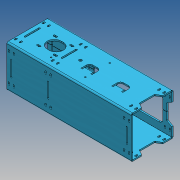
# Autodesk Inventor part: Pliegue Principal
Saved by Autodesk Inventor 2017 (Build 210142000, 142)
## iProperties
Part Number: Pliegue Principal
Material: Genérico
Document SubType Name: Chapa
Designer: Leo
Density: 1 g/cm^3
Appearance: Turquesa
Sheet Metal Rule: Por defecto
Sheet Metal Width: 355,000 mm
Sheet Metal Length: 458,387 mm
Sheet Metal Area: 162727,287 mm^2
Flat Pattern Width: 35.5 cm
Flat Pattern Length: 45.8387 cm
Flat Pattern Area: 1627.27 cm^2
Author: Leo
Autodesk Inventor part; units mm, degrees
ref_plane "YZ Plane" through (0, 0, 0) normal (1, 0, 0) x (0, 1, 0)
ref_plane "XZ Plane" through (0, 0, 0) normal (0, 1, 0) x (-1, 0, 0)
ref_plane "XY Plane" through (0, 0, 0) normal (0, 0, 1) x (1, 0, 0)
sketch "Boceto1" plane through (0, 0, 0) normal (0, 0, 1) x (1, 0, 0)
  circle A0 centre (0, 0) radius 4.805 construction
  circle A1 centre (0, 0) radius 22 construction
  circle A2 centre (72, 0) radius 50 construction
  line L0 (28.2, 28.2) -> (-28.2, 28.2) construction
  line L1 (-28.2, 28.2) -> (-28.2, -28.2) construction
  line L2 (-28.2, -28.2) -> (28.2, -28.2) construction
  line L3 (28.2, -28.2) -> (28.2, 28.2) construction
  line L4 (-8.5556, 20.2683) -> (52.5556, 46.0642) construction
  line L5 (52.5556, -46.0642) -> (-8.5556, -20.2683) construction
  line L6 (51.8, -14) -> (251.8, -14) construction
  line L7 (251.8, -14) -> (251.8, -56) construction
  line L8 (251.8, -56) -> (51.8, -56) construction
  line L9 (51.8, -56) -> (51.8, -14) construction
  circle A3 centre (72, 0) radius 4
  line L10 (-20.57, 21.07) -> (-26.57, 21.07)
  arc A4 (-26.57, 26.07) -> (-26.57, 21.07) centre (-26.57, 23.57) ccw
  line L11 (-26.57, 26.07) -> (-20.57, 26.07)
  arc A5 (-20.57, 21.07) -> (-20.57, 26.07) centre (-20.57, 23.57) ccw
  line L12 (20.57, -21.07) -> (26.57, -21.07)
  arc A6 (26.57, -26.07) -> (26.57, -21.07) centre (26.57, -23.57) ccw
  line L13 (26.57, -26.07) -> (20.57, -26.07)
  arc A7 (20.57, -21.07) -> (20.57, -26.07) centre (20.57, -23.57) ccw
  line L14 (20.57, 26.07) -> (26.57, 26.07)
  arc A8 (26.57, 21.07) -> (26.57, 26.07) centre (26.57, 23.57) ccw
  line L15 (26.57, 21.07) -> (20.57, 21.07)
  arc A9 (20.57, 26.07) -> (20.57, 21.07) centre (20.57, 23.57) ccw
  line L16 (-20.57, 23.57) -> (-26.57, 23.57) construction
  line L17 (20.57, 23.57) -> (26.57, 23.57) construction
  line L18 (48.6318, 0) -> (95.3682, 0) construction
  circle A10 centre (120.734, 35) radius 2
  circle A11 centre (120.734, -35) radius 2
  circle A12 centre (120.734, 35) radius 10 construction
  circle A13 centre (72, 0) radius 30 construction
  line L19 (119.667, 25.0571) -> (75.2009, 29.8287) construction
  line L20 (-78.2, 60) -> (276.8, 60)
  line L21 (276.8, 60) -> (276.8, -60)
  line L22 (276.8, -60) -> (-78.2, -60)
  line L23 (-78.2, -60) -> (-78.2, 60)
  circle A14 centre (23.266, -35) radius 2
  circle A15 centre (23.266, -35) radius 10 construction
  circle A16 centre (72, 0) radius 11 construction
  line L24 (-26.57, -21.07) -> (-20.57, -21.07)
  arc A17 (-20.57, -26.07) -> (-20.57, -21.07) centre (-20.57, -23.57) ccw
  line L25 (-20.57, -26.07) -> (-26.57, -26.07)
  arc A18 (-26.57, -21.07) -> (-26.57, -26.07) centre (-26.57, -23.57) ccw
  line L26 (-26.57, -23.57) -> (-20.57, -23.57) construction
  line L27 (-23.57, -23.57) -> (-23.57, 23.57) construction
  line L28 (23.57, 23.57) -> (23.57, -18.9602) construction
  line L29 (-23.57, 0) -> (23.57, 0) construction
  line L30 (-3, -20) -> (3, -20)
  arc A19 (3, -20) -> (3, 20) centre (3, 0) ccw
  line L31 (3, 20) -> (-3, 20)
  arc A20 (-3, 20) -> (-3, -20) centre (-3, 0) ccw
  line L32 (-67.9, 20.5) -> (-67.9, -20.5)
  arc A21 (-67.9, -20.5) -> (-63.5, -20.5) centre (-65.7, -20.5) ccw
  line L33 (-63.5, -20.5) -> (-63.5, 20.5)
  arc A22 (-63.5, 20.5) -> (-67.9, 20.5) centre (-65.7, 20.5) ccw
  line L34 (266.5, 20.5) -> (266.5, -20.5)
  arc A23 (262.1, -20.5) -> (266.5, -20.5) centre (264.3, -20.5) ccw
  line L35 (262.1, -20.5) -> (262.1, 20.5)
  arc A24 (266.5, 20.5) -> (262.1, 20.5) centre (264.3, 20.5) ccw
  line L36 (99.3, 60) -> (99.3, -60) construction
  line L37 (37.8, 20.5) -> (37.8, -20.5)
  arc A25 (37.8, -20.5) -> (42.2, -20.5) centre (40, -20.5) ccw
  line L38 (42.2, -20.5) -> (42.2, 20.5)
  arc A26 (42.2, 20.5) -> (37.8, 20.5) centre (40, 20.5) ccw
  line L39 (42.2, 0) -> (37.8, 0) construction
  line L40 (40, -20.5) -> (40, 20.5) construction
  line L41 (92.15, -19) -> (92.15, -3)
  arc A27 (101.15, 6) -> (92.15, -3) centre (101.15, -3) ccw
  line L42 (101.15, 6) -> (115.15, 6)
  arc A28 (124.15, -3) -> (115.15, 6) centre (115.15, -3) ccw
  line L43 (124.15, -3) -> (124.15, -19)
  line L44 (120.15, -19) -> (120.15, -3)
  arc A29 (120.15, -3) -> (115.15, 2) centre (115.15, -3) ccw
  line L45 (115.15, 2) -> (101.15, 2)
  arc A30 (101.15, 2) -> (96.15, -3) centre (101.15, -3) ccw
  line L46 (96.15, -3) -> (96.15, -19)
  line L47 (120.15, -19) -> (124.15, -19)
  line L48 (96.15, -19) -> (92.15, -19)
  circle A31 centre (108.15, -4) radius 1.5
  line L49 (120.15, -10) -> (96.15, -10) construction
  line L50 (152.15, 24.7694) -> (152.15, -40.3489) construction
  line L51 (212.15, -19) -> (212.15, -3)
  arc A32 (212.15, -3) -> (203.15, 6) centre (203.15, -3) ccw
  line L52 (203.15, 6) -> (189.15, 6)
  arc A33 (189.15, 6) -> (180.15, -3) centre (189.15, -3) ccw
  line L53 (180.15, -3) -> (180.15, -19)
  line L54 (184.15, -19) -> (184.15, -3)
  arc A34 (189.15, 2) -> (184.15, -3) centre (189.15, -3) ccw
  line L55 (189.15, 2) -> (203.15, 2)
  arc A35 (208.15, -3) -> (203.15, 2) centre (203.15, -3) ccw
  line L56 (208.15, -3) -> (208.15, -19)
  line L57 (184.15, -19) -> (180.15, -19)
  line L58 (208.15, -19) -> (212.15, -19)
  circle A36 centre (196.15, -4) radius 1.5
  line L59 (184.15, -10) -> (208.15, -10) construction
  line L60 (-72.9, 44.2) -> (-72.9, 35.8) construction
  line L61 (-75.1, 42) -> (-75.1, 38)
  line L62 (-70.7, 38) -> (-70.7, 42)
  arc A37 (-70.7, 42) -> (-75.1, 42) centre (-72.9, 42) ccw
  arc A38 (-75.1, 38) -> (-70.7, 38) centre (-72.9, 38) ccw
  line L63 (-58.5, 44.2) -> (-58.5, 35.8) construction
  line L64 (-60.7, 42) -> (-60.7, 38)
  line L65 (-56.3, 38) -> (-56.3, 42)
  arc A39 (-56.3, 42) -> (-60.7, 42) centre (-58.5, 42) ccw
  arc A40 (-60.7, 38) -> (-56.3, 38) centre (-58.5, 38) ccw
  line L66 (-65.7, 20.5) -> (-65.7, -20.5) construction
  line L67 (-72.9, -44.2) -> (-72.9, -35.8) construction
  line L68 (-75.1, -42) -> (-75.1, -38)
  line L69 (-70.7, -38) -> (-70.7, -42)
  arc A41 (-75.1, -42) -> (-70.7, -42) centre (-72.9, -42) ccw
  arc A42 (-70.7, -38) -> (-75.1, -38) centre (-72.9, -38) ccw
  line L70 (-58.5, -44.2) -> (-58.5, -35.8) construction
  line L71 (-60.7, -42) -> (-60.7, -38)
  line L72 (-56.3, -38) -> (-56.3, -42)
  arc A43 (-60.7, -42) -> (-56.3, -42) centre (-58.5, -42) ccw
  arc A44 (-56.3, -38) -> (-60.7, -38) centre (-58.5, -38) ccw
  line L73 (273.7, 42) -> (273.7, 38)
  line L74 (269.3, 38) -> (269.3, 42)
  arc A45 (273.7, 42) -> (269.3, 42) centre (271.5, 42) ccw
  arc A46 (269.3, 38) -> (273.7, 38) centre (271.5, 38) ccw
  line L75 (259.3, 42) -> (259.3, 38)
  line L76 (254.9, 38) -> (254.9, 42)
  arc A47 (259.3, 42) -> (254.9, 42) centre (257.1, 42) ccw
  arc A48 (254.9, 38) -> (259.3, 38) centre (257.1, 38) ccw
  arc A49 (273.7, -38) -> (269.3, -38) centre (271.5, -38) ccw
  arc A50 (259.3, -38) -> (254.9, -38) centre (257.1, -38) ccw
  line L77 (259.3, -42) -> (259.3, -38)
  line L78 (269.3, -38) -> (269.3, -42)
  line L79 (254.9, -38) -> (254.9, -42)
  arc A51 (254.9, -42) -> (259.3, -42) centre (257.1, -42) ccw
  arc A52 (269.3, -42) -> (273.7, -42) centre (271.5, -42) ccw
  line L80 (273.7, -42) -> (273.7, -38)
  line L81 (-12.85, 67.9795) -> (-12.85, -73.496) construction
  line L82 (49.4, 42) -> (49.4, 38)
  line L83 (45, 38) -> (45, 42)
  arc A53 (49.4, 42) -> (45, 42) centre (47.2, 42) ccw
  arc A54 (45, 38) -> (49.4, 38) centre (47.2, 38) ccw
  line L84 (35, 42) -> (35, 38)
  line L85 (30.6, 38) -> (30.6, 42)
  arc A55 (35, 42) -> (30.6, 42) centre (32.8, 42) ccw
  arc A56 (30.6, 38) -> (35, 38) centre (32.8, 38) ccw
  arc A57 (49.4, -38) -> (45, -38) centre (47.2, -38) ccw
  arc A58 (35, -38) -> (30.6, -38) centre (32.8, -38) ccw
  line L86 (35, -42) -> (35, -38)
  line L87 (45, -38) -> (45, -42)
  line L88 (30.6, -38) -> (30.6, -42)
  arc A59 (30.6, -42) -> (35, -42) centre (32.8, -42) ccw
  arc A60 (45, -42) -> (49.4, -42) centre (47.2, -42) ccw
  line L89 (49.4, -42) -> (49.4, -38)
  line L90 (276.8, 30.2572) -> (263.2, 22.4053)
  line L91 (276.8, -30.2572) -> (263.2, -22.4053)
  point P0 (-28.2, 0)
  point P1 (0, -28.2)
  point P2 (276.8, 0)
  point P3 (0, 20)
  point P4 (-67.9, 0)
  point P5 (-78.2, 0)
  point P6 (40, 0)
  point P7 (108.15, 2)
  point P8 (-72.9, 40)
  point P9 (-58.5, 40)
  point P10 (-72.9, -40)
  point P11 (-58.5, -40)
  point P12 (32.8, 44.2)
  dimension "d15" = 20
  dimension "d17" = 60
  dimension "d29" = 4
  dimension "d1" = 56.4
  dimension "d2" = 72
  dimension "d4" = 200
  dimension "d5" = 42
  dimension "d6" = 8
  dimension "d8" = 5
  dimension "d9" = 41.14
  dimension "d10" = 6
  dimension "d11" = 53.14
  dimension "d12" = 6
  dimension "d13" = 4
  dimension "d14" = 100
  dimension "d16" = 70
  dimension "d18" = 4
  dimension "d19" = 33.93
  dimension "d20" = 22
  dimension "d21" = 120
  dimension "d22" = 130
  dimension "d23" = 20
  dimension "d42" = 47.14
  dimension "d43" = 47.14
  dimension "d44" = 20
  dimension "d45" = 6
  dimension "d46" = 14.2
  dimension "d47" = 25
  dimension "d62" = 4.4
  dimension "d63" = 41
  dimension "d70" = 4.4
  dimension "d86" = 50
  dimension "d87" = 355
  dimension "d88" = 12.5
  dimension "d89" = 12.5
  dimension "d90" = 23.6
  dimension "d91" = 11.8
  dimension "d97" = 190.1
  dimension "d118" = 4
  dimension "d119" = 5
  dimension "d120" = 3
  dimension "d121" = 4
  dimension "d122" = 5
  dimension "d123" = 12
  dimension "d124" = 6
  dimension "d125" = 24
  dimension "d126" = 120
  dimension "d142" = 10
  dimension "d143" = 4
  dimension "d144" = 80
  dimension "d145" = 5
  dimension "d146" = 60
  constraints: 193 end point, 111 point on circle, 82 symmetric about line, 59 centre point, 52 tangent, 20 midpoint, 18 parallel, 17 point on line, 13 horizontal alignment, 11 vertical, 10 horizontal, 8 coincident, 8 equal radius, 8 perpendicular, 6 vertical alignment, 4 collinear, 4 equal length, 1 concentric, 42 other
  measures "d1" distance of L0.end L1.end
  measures "d2" distance of A2.centre point (0, 0)
  measures "d4" distance of L7.end L8.end
  measures "d5" distance of L6.end L7.end
  measures "d6" diameter of A3
  measures "d8" distance between parallel lines of L11 L10
  measures "d9" distance of L17.start L16.start
  measures "d10" distance of L16.start L16.end
  measures "d11" distance of L17.end L16.end
  measures "d12" distance of L16.start L16.end
  measures "d13" diameter of A10
  measures "d14" diameter of A2
  measures "d16" distance of point (120.734, 35) A11.centre
  measures "d18" distance between parallel lines of L22 L8
  measures "d19" distance edge to line of A4 L20
  measures "d20" diameter of A16
  measures "d21" distance of L20.end L21.end
  measures "d22" distance between parallel lines of L23 L9
  measures "d23" diameter of A15
  measures "d42" distance from line of L26.start L16
  measures "d43" distance between parallel lines of L28 L27
  measures "d44" radius of A20
  measures "d45" distance of L30.start L30.end
  measures "d46" distance between parallel lines of L2 L6
  measures "d47" distance between parallel lines of L21 L7
  measures "d62" distance between parallel lines of L33 L32
  measures "d63" distance of L32.start L32.end
  measures "d70" distance between parallel lines of L35 L34
  measures "d86" distance between parallel lines of L23 L1
  measures "d87" distance of L20.start L20.end
  measures "d88" distance from line of L66.start L23
  measures "d89" distance from line of A24.centre L21
  measures "d90" distance between parallel lines of L3 L9
  measures "d91" distance from line of L40.start L3
  measures "d97" distance from line of L35 A2.centre
  measures "d118" distance between parallel lines of L41 L46
  measures "d119" radius of A30
  measures "d120" diameter of A31
  measures "d121" distance between parallel lines of L49 L6
  measures "d122" distance between parallel lines of L6 L47
  measures "d123" distance between parallel lines of L45 L49
  measures "d124" distance from line of L45 A31.centre
  measures "d125" distance between parallel lines of L44 L46
  measures "d126" distance between parallel lines of L51 L41
  measures "d142" distance between parallel lines of L64 L62
  measures "d143" distance of L61.start L61.end
  measures "d144" diameter of point (-72.9, 40) L18
  measures "d145" distance between parallel lines of L83 L40
  measures "d146" angle of L90 L91
extrude "Extrusión1" add sketch "Boceto1" along normal blind 4 contours L20 L21 L90 A24 L35 A23 L91 L22 L23
sketch "Boceto2" plane through (-78.2, -56, 4) normal (0, -1, 0) x (1, 0, 0)
  line L0 (355, 0) -> (0, 0)
  line L1 (0, 0) -> (0, -120)
  line L2 (0, -120) -> (355, -120)
  line L3 (355, -120) -> (355, 0)
  constraints: 6 end point, 1 horizontal, 1 perpendicular, 1 vertical
edge flange "Pestaña1" height 120 angle 90 thickness 4 bend radius 0.1 thickness toward (0, -1, 0) relief tear relief width 4 relief depth 2 edges at (99.3, -60, 0) wall of the first edge with corners at (276.8, -56, 4) (-78.2, -56, 4) (-78.2, -56, -116) (276.8, -56, -116)
bend "Doblez1"
corner "Esquina1"
fold "Pliegue1" angle 90 bend radius 1 thickness 4 k factor 0.44 line from (120.15, -10, 0) to (96.15, -10, 0) line at bend centre moving side (0, 1, 0) folds toward (0, 0, -1)
fold "Pliegue2" angle 90 bend radius 0.1 thickness 4 k factor 0.44 line from (184.15, -10, 0) to (208.15, -10, 0) line at bend centre moving side (0, 1, 0) folds toward (0, 0, -1)
sketch "Boceto4" plane through (-78.2, 60, 0) normal (0, 1, 0) x (1, 0, 0)
  line L0 (355, 116) -> (0, 116)
  line L1 (0, 0) -> (355, 0)
  line L2 (0, 116) -> (0, 56.25)
  line L3 (0, 56.25) -> (130.8, 56.25)
  line L4 (130.8, 56.25) -> (130.8, 80)
  arc A0 (142.8, 92) -> (130.8, 80) centre (142.8, 80) ccw
  line L5 (142.8, 92) -> (318, 92)
  arc A1 (330, 80) -> (318, 92) centre (318, 80) ccw
  line L6 (330, 80) -> (330, 56.25)
  line L7 (330, 56.25) -> (340.4, 56.25)
  line L8 (355, 116) -> (355, 86.1417)
  line L9 (355, 0) -> (355, 25.8583)
  line L10 (340.4, 55.75) -> (330, 55.75)
  line L11 (330, 55.75) -> (330, 32)
  arc A2 (318, 20) -> (330, 32) centre (318, 32) ccw
  line L12 (318, 20) -> (142.8, 20)
  arc A3 (130.8, 32) -> (142.8, 20) centre (142.8, 32) ccw
  line L13 (130.8, 32) -> (130.8, 55.75)
  line L14 (130.8, 55.75) -> (0, 55.75)
  line L15 (0, 55.75) -> (0, 0)
  arc A4 (341.45, 78.3187) -> (340.4, 76.5) centre (342.5, 76.5) ccw
  line L16 (340.4, 76.5) -> (340.4, 35.5)
  arc A5 (340.4, 35.5) -> (341.45, 33.6813) centre (342.5, 35.5) ccw
  line L17 (10.4, 35.5) -> (10.4, 76.5)
  arc A6 (14.6, 76.5) -> (10.4, 76.5) centre (12.5, 76.5) ccw
  line L18 (14.6, 76.5) -> (14.6, 35.5)
  arc A7 (10.4, 35.5) -> (14.6, 35.5) centre (12.5, 35.5) ccw
  line L19 (343.659, 56) -> (340.4, 56) construction
  line L20 (65.25, -49.8772) -> (65.25, 182.1295) construction
  line L21 (5.4, 11.9) -> (5.4, 20.1) construction
  line L22 (7.5, 14) -> (7.5, 18)
  line L23 (3.3, 18) -> (3.3, 14)
  arc A8 (3.3, 14) -> (7.5, 14) centre (5.4, 14) ccw
  arc A9 (7.5, 18) -> (3.3, 18) centre (5.4, 18) ccw
  line L24 (12.5, 35.5) -> (12.5, 76.5) construction
  line L25 (10.4, 56) -> (14.6, 56) construction
  line L26 (17.5, 14) -> (17.5, 18)
  line L27 (21.7, 18) -> (21.7, 14)
  arc A10 (17.5, 14) -> (21.7, 14) centre (19.6, 14) ccw
  arc A11 (21.7, 18) -> (17.5, 18) centre (19.6, 18) ccw
  line L28 (7.5, 98) -> (7.5, 94)
  line L29 (3.3, 94) -> (3.3, 98)
  arc A12 (7.5, 98) -> (3.3, 98) centre (5.4, 98) ccw
  arc A13 (3.3, 94) -> (7.5, 94) centre (5.4, 94) ccw
  arc A14 (21.7, 98) -> (17.5, 98) centre (19.6, 98) ccw
  arc A15 (17.5, 94) -> (21.7, 94) centre (19.6, 94) ccw
  line L30 (21.7, 94) -> (21.7, 98)
  line L31 (17.5, 98) -> (17.5, 94)
  line L32 (123, 14) -> (123, 18)
  line L33 (127.2, 18) -> (127.2, 14)
  arc A16 (123, 14) -> (127.2, 14) centre (125.1, 14) ccw
  arc A17 (127.2, 18) -> (123, 18) centre (125.1, 18) ccw
  arc A18 (108.8, 14) -> (113, 14) centre (110.9, 14) ccw
  arc A19 (113, 18) -> (108.8, 18) centre (110.9, 18) ccw
  line L34 (108.8, 18) -> (108.8, 14)
  line L35 (113, 14) -> (113, 18)
  arc A20 (113, 98) -> (108.8, 98) centre (110.9, 98) ccw
  line L36 (113, 98) -> (113, 94)
  line L37 (108.8, 94) -> (108.8, 98)
  arc A21 (108.8, 94) -> (113, 94) centre (110.9, 94) ccw
  arc A22 (123, 94) -> (127.2, 94) centre (125.1, 94) ccw
  line L38 (123, 98) -> (123, 94)
  arc A23 (127.2, 98) -> (123, 98) centre (125.1, 98) ccw
  line L39 (127.2, 94) -> (127.2, 98)
  line L40 (120.1, 35.5) -> (120.1, 76.5)
  arc A24 (120.1, 76.5) -> (115.9, 76.5) centre (118, 76.5) ccw
  line L41 (115.9, 76.5) -> (115.9, 35.5)
  arc A25 (115.9, 35.5) -> (120.1, 35.5) centre (118, 35.5) ccw
  line L42 (230.25, 152.4167) -> (230.25, -55.455) construction
  line L43 (333.3, 94) -> (333.3, 98)
  arc A26 (337.5, 98) -> (333.3, 98) centre (335.4, 98) ccw
  line L44 (337.5, 98) -> (337.5, 94)
  arc A27 (333.3, 94) -> (337.5, 94) centre (335.4, 94) ccw
  line L45 (347.5, 98) -> (347.5, 94)
  arc A28 (351.7, 98) -> (347.5, 98) centre (349.6, 98) ccw
  line L46 (351.7, 94) -> (351.7, 98)
  arc A29 (347.5, 94) -> (351.7, 94) centre (349.6, 94) ccw
  arc A30 (333.3, 14) -> (337.5, 14) centre (335.4, 14) ccw
  line L47 (333.3, 18) -> (333.3, 14)
  arc A31 (337.5, 18) -> (333.3, 18) centre (335.4, 18) ccw
  line L48 (337.5, 14) -> (337.5, 18)
  line L49 (347.5, 14) -> (347.5, 18)
  arc A32 (351.7, 18) -> (347.5, 18) centre (349.6, 18) ccw
  line L50 (351.7, 18) -> (351.7, 14)
  arc A33 (347.5, 14) -> (351.7, 14) centre (349.6, 14) ccw
  line L51 (355, 86.1417) -> (341.45, 78.3187)
  line L52 (355, 116) -> (355, 0.1) projected
  line L53 (355, 25.8583) -> (341.45, 33.6813)
  point P0 (342.5, 55.75)
  point P1 (342.0295, 56)
  point P2 (120.4, 0)
  point P3 (5.4, 16)
  dimension "d58" = 0.5
  dimension "d59" = 0.5
  dimension "d60" = 20
  dimension "d61" = 24
  dimension "d71" = 130.8
  dimension "d72" = 25
  dimension "d102" = 12
  dimension "d103" = 0.25
  dimension "d109" = 12.5
  dimension "d148" = 10.4
  dimension "d149" = 10.4
  dimension "d150" = 4
  dimension "d151" = 80
  dimension "d152" = 105.5
  dimension "d153" = 10
  dimension "d154" = 5
  dimension "d155" = 60
  dimension "d156" = 41
  dimension "d157" = 4.2
  dimension "d158" = 12.5
  constraints: 108 end point, 72 symmetric about line, 70 point on circle, 34 centre point, 20 tangent, 10 perpendicular, 9 vertical, 6 equal radius, 6 point on line, 5 midpoint, 4 coincident, 3 collinear, 3 parallel, 2 equal length, 1 horizontal alignment, 1 vertical alignment, 25 other
  measures "d58" distance between parallel lines of L10 L7
  measures "d59" distance between parallel lines of L14 L3
  measures "d60" distance between parallel lines of L1 L12
  measures "d61" distance between parallel lines of L0 L5
  measures "d71" distance between parallel lines of L15 L13
  measures "d72" distance between parallel lines of L8 L6
  measures "d102" radius of A0
  measures "d103" distance between parallel lines of L10 L19
  measures "d109" distance from line of L24.end L2
  measures "d148" distance between parallel lines of L17 L15
  measures "d149" distance from line of point (120.4, 0) L13
  measures "d150" distance of L23.start L23.end
  measures "d151" diameter of point (5.4, 16) L25
  measures "d152" distance from line of A25.centre L24
  measures "d153" distance between parallel lines of L22 L26
  measures "d154" distance from line of L49 A5.centre
  measures "d155" angle of L51 L53
  measures "d156" distance of L18.start L18.end
  measures "d157" distance between parallel lines of L18 L17
  measures "d158" distance from line of A4.centre L52
sheet face with bend "Cara1" sketch "Boceto4" thickness 4 toward (0, -1, 0) bend radius 0.1 relief tear relief width 4 relief depth 2 contours L8 L51 A4 L16 L7 L6 A1 L5 A0 L4 L3 L40 A24 L41 L18 A6 L17 L2 L0 | L17 A6 L18 L3 | L41 A24 L40 L3
bend "Doblez2"
sheet face with bend "Cara2" sketch "Boceto4" thickness 4 toward (0, -1, 0) bend radius 0.1 relief tear relief width 4 relief depth 2 contours L9 L1 L15 L14 L17 A7 L18 L41 A25 L40 L13 A3 L12 A2 L11 L10 L16 A5 L53 | L14 L18 A7 L17 | L14 L40 A25 L41
bend "Doblez3"
extrude "Extrusión4" cut sketch "Boceto4" against normal blind 10 contours L17 A6 L18 L3 | L3 L18 L14 L17 | L14 L18 A7 L17 | L41 A24 L40 L3 | L3 L40 L14 L41 | L14 L40 A25 L41 | A8 L23 A9 L22 | L26 A11 L27 A10 | L32 A17 L33 A16 | L34 A19 L35 A18 | L47 A31 L48 A30 | L49 A32 L50 A33
sketch "Boceto5" plane through (276.8, 60, -116) normal (0, 0, -1) x (-1, 0, 0)
  line L0 (0, -4) -> (355, -4) projected
  line L1 (0, -116) -> (355, -116) projected
  line L2 (355, 0) -> (355, -4) projected
  line L3 (355, -4) -> (355, -116)
  line L4 (0, -116) -> (0, -4)
  line L5 (344.7, -80.5) -> (344.7, -39.5) projected
  arc A0 (344.7, -39.5) -> (340.3, -39.5) centre (342.5, -39.5) ccw projected
  line L6 (340.3, -39.5) -> (340.3, -80.5) projected
  arc A1 (340.3, -80.5) -> (344.7, -80.5) centre (342.5, -80.5) ccw projected
  line L7 (355, 0) -> (355, -115.9) projected
  line L8 (355, -57.95) -> (321.347, -57.95)
  line L9 (234.6, -39.5) -> (234.6, -80.5) projected
  arc A2 (239, -39.5) -> (234.6, -39.5) centre (236.8, -39.5) ccw projected
  line L10 (239, -80.5) -> (239, -39.5) projected
  arc A3 (234.6, -80.5) -> (239, -80.5) centre (236.8, -80.5) ccw projected
  line L11 (14.7, -80.5) -> (14.7, -39.5) projected
  arc A4 (14.7, -39.5) -> (14.7, -39.5) centre (12.5, -39.5) ccw projected
  arc A5 (14.7, -80.5) -> (14.7, -80.5) centre (12.5, -80.5) ccw projected
  line L12 (73.65, -54) -> (87.65, -54) projected
  arc A6 (96.65, -63) -> (87.65, -54) centre (87.65, -63) ccw projected
  line L13 (96.65, -63) -> (96.65, -79) projected
  line L14 (92.65, -79) -> (96.65, -79) projected
  line L15 (92.65, -79) -> (92.65, -63) projected
  arc A7 (92.65, -63) -> (87.65, -58) centre (87.65, -63) ccw projected
  line L16 (87.65, -58) -> (73.65, -58) projected
  arc A8 (73.65, -58) -> (68.65, -63) centre (73.65, -63) ccw projected
  arc A9 (73.65, -54) -> (64.65, -63) centre (73.65, -63) ccw projected
  line L17 (64.65, -79) -> (64.65, -63) projected
  line L18 (68.65, -63) -> (68.65, -79) projected
  line L19 (68.65, -79) -> (64.65, -79) projected
  line L20 (156.65, -79) -> (152.65, -79) projected
  line L21 (152.65, -79) -> (152.65, -63) projected
  line L22 (156.65, -79) -> (156.65, -63) projected
  arc A10 (161.65, -58) -> (156.65, -63) centre (161.65, -63) ccw projected
  arc A11 (161.65, -54) -> (152.65, -63) centre (161.65, -63) ccw projected
  line L23 (161.65, -54) -> (175.65, -54) projected
  line L24 (161.65, -58) -> (175.65, -58) projected
  arc A12 (180.65, -63) -> (175.65, -58) centre (175.65, -63) ccw projected
  arc A13 (184.65, -63) -> (175.65, -54) centre (175.65, -63) ccw projected
  line L25 (184.65, -63) -> (184.65, -79) projected
  line L26 (184.65, -79) -> (180.65, -79) projected
  line L27 (180.65, -63) -> (180.65, -79) projected
  line L28 (254.3, -15) -> (299.3, -15)
  line L29 (304.3, -20) -> (304.3, -100)
  line L30 (299.3, -105) -> (254.3, -105)
  line L31 (249.3, -100) -> (249.3, -20)
  arc A14 (254.3, -15) -> (249.3, -20) centre (254.3, -20) ccw
  arc A15 (304.3, -20) -> (299.3, -15) centre (299.3, -20) ccw
  arc A16 (299.3, -105) -> (304.3, -100) centre (299.3, -100) ccw
  arc A17 (249.3, -100) -> (254.3, -105) centre (254.3, -100) ccw
  circle A18 centre (80.65, -64) radius 1.5 projected
  circle A19 centre (168.65, -64) radius 1.5 projected
  line L32 (13.6, -37.5947) -> (0, -29.7428) projected
  line L33 (0, -29.7428) -> (0, -4.1) projected
  line L34 (13.6, -37.5947) -> (0, -29.7428) projected
  arc A20 (14.7, -39.5) -> (13.6, -37.5947) centre (12.5, -39.5) ccw projected
  line L35 (14.7, -80.5) -> (14.7, -39.5) projected
  arc A21 (13.6, -82.4053) -> (14.7, -80.5) centre (12.5, -80.5) ccw projected
  line L36 (0, -90.2572) -> (13.6, -82.4053) projected
  line L37 (0, -115.9) -> (0, -90.2572) projected
  line L38 (0, -115.9) -> (355, -115.9) projected
  line L39 (355, -4.1) -> (355, -115.9) projected
  line L40 (92.65, -71.4608) -> (68.65, -71.4608) projected
  line L41 (68.65, -71.4608) -> (68.65, -79) projected
  line L42 (68.65, -79) -> (64.65, -79) projected
  line L43 (64.65, -79) -> (64.65, -63) projected
  arc A22 (73.65, -54) -> (64.65, -63) centre (73.65, -63) ccw projected
  line L44 (73.65, -54) -> (87.65, -54) projected
  arc A23 (96.65, -63) -> (87.65, -54) centre (87.65, -63) ccw projected
  line L45 (96.65, -63) -> (96.65, -79) projected
  line L46 (96.65, -79) -> (92.65, -79) projected
  line L47 (92.65, -79) -> (92.65, -71.4608) projected
  arc A24 (279.8, -80) -> (279.8, -40) centre (279.8, -60) ccw projected
  line L48 (279.8, -80) -> (273.8, -80) projected
  arc A25 (273.8, -40) -> (273.8, -80) centre (273.8, -60) ccw projected
  line L49 (273.8, -40) -> (279.8, -40) projected
  line L50 (180.65, -72.1677) -> (156.65, -72.1677) projected
  line L51 (156.65, -72.1677) -> (156.65, -79) projected
  line L52 (156.65, -79) -> (152.65, -79) projected
  line L53 (152.65, -79) -> (152.65, -63) projected
  arc A26 (161.65, -54) -> (152.65, -63) centre (161.65, -63) ccw projected
  line L54 (161.65, -54) -> (175.65, -54) projected
  arc A27 (184.65, -63) -> (175.65, -54) centre (175.65, -63) ccw projected
  line L55 (184.65, -63) -> (184.65, -79) projected
  line L56 (184.65, -79) -> (180.65, -79) projected
  line L57 (180.65, -79) -> (180.65, -72.1677) projected
  arc A28 (239, -39.5) -> (234.6, -39.5) centre (236.8, -39.5) ccw projected
  line L58 (239, -39.5) -> (239, -80.5) projected
  arc A29 (234.6, -80.5) -> (239, -80.5) centre (236.8, -80.5) ccw projected
  line L59 (234.6, -80.5) -> (234.6, -39.5) projected
  arc A30 (344.7, -39.5) -> (340.3, -39.5) centre (342.5, -39.5) ccw projected
  line L60 (344.7, -39.5) -> (344.7, -80.5) projected
  arc A31 (340.3, -80.5) -> (344.7, -80.5) centre (342.5, -80.5) ccw projected
  line L61 (340.3, -80.5) -> (340.3, -39.5) projected
  circle A32 centre (204.8, -60) radius 4 projected
  arc A33 (297.37, -81.07) -> (297.37, -86.07) centre (297.37, -83.57) ccw projected
  line L62 (297.37, -81.07) -> (303.37, -81.07) projected
  arc A34 (303.37, -86.07) -> (303.37, -81.07) centre (303.37, -83.57) ccw projected
  line L63 (303.37, -86.07) -> (297.37, -86.07) projected
  arc A35 (250.23, -33.93) -> (250.23, -38.93) centre (250.23, -36.43) ccw projected
  line L64 (250.23, -33.93) -> (256.23, -33.93) projected
  arc A36 (256.23, -38.93) -> (256.23, -33.93) centre (256.23, -36.43) ccw projected
  line L65 (256.23, -38.93) -> (250.23, -38.93) projected
  arc A37 (250.23, -81.07) -> (250.23, -86.07) centre (250.23, -83.57) ccw projected
  line L66 (250.23, -81.07) -> (256.23, -81.07) projected
  arc A38 (256.23, -86.07) -> (256.23, -81.07) centre (256.23, -83.57) ccw projected
  line L67 (256.23, -86.07) -> (250.23, -86.07) projected
  arc A39 (303.37, -38.93) -> (303.37, -33.93) centre (303.37, -36.43) ccw projected
  line L68 (303.37, -38.93) -> (297.37, -38.93) projected
  arc A40 (297.37, -33.93) -> (297.37, -38.93) centre (297.37, -36.43) ccw projected
  line L69 (297.37, -33.93) -> (303.37, -33.93) projected
  arc A41 (17.5, -102) -> (21.9, -102) centre (19.7, -102) ccw projected
  line L70 (17.5, -102) -> (17.5, -98) projected
  arc A42 (21.9, -98) -> (17.5, -98) centre (19.7, -98) ccw projected
  line L71 (21.9, -98) -> (21.9, -102) projected
  arc A43 (3.1, -102) -> (7.5, -102) centre (5.3, -102) ccw projected
  line L72 (3.1, -102) -> (3.1, -98) projected
  arc A44 (7.5, -98) -> (3.1, -98) centre (5.3, -98) ccw projected
  line L73 (7.5, -98) -> (7.5, -102) projected
  arc A45 (17.5, -22) -> (21.9, -22) centre (19.7, -22) ccw projected
  line L74 (17.5, -22) -> (17.5, -18) projected
  arc A46 (21.9, -18) -> (17.5, -18) centre (19.7, -18) ccw projected
  line L75 (21.9, -18) -> (21.9, -22) projected
  arc A47 (3.1, -22) -> (7.5, -22) centre (5.3, -22) ccw projected
  line L76 (3.1, -22) -> (3.1, -18) projected
  arc A48 (7.5, -18) -> (3.1, -18) centre (5.3, -18) ccw projected
  line L77 (7.5, -18) -> (7.5, -22) projected
  arc A49 (241.8, -102) -> (246.2, -102) centre (244, -102) ccw projected
  line L78 (241.8, -102) -> (241.8, -98) projected
  arc A50 (246.2, -98) -> (241.8, -98) centre (244, -98) ccw projected
  line L79 (246.2, -98) -> (246.2, -102) projected
  arc A51 (227.4, -102) -> (231.8, -102) centre (229.6, -102) ccw projected
  line L80 (227.4, -102) -> (227.4, -98) projected
  arc A52 (231.8, -98) -> (227.4, -98) centre (229.6, -98) ccw projected
  line L81 (231.8, -98) -> (231.8, -102) projected
  arc A53 (246.2, -18) -> (241.8, -18) centre (244, -18) ccw projected
  line L82 (246.2, -18) -> (246.2, -22) projected
  arc A54 (241.8, -22) -> (246.2, -22) centre (244, -22) ccw projected
  line L83 (241.8, -22) -> (241.8, -18) projected
  arc A55 (227.4, -22) -> (231.8, -22) centre (229.6, -22) ccw projected
  line L84 (227.4, -22) -> (227.4, -18) projected
  arc A56 (231.8, -18) -> (227.4, -18) centre (229.6, -18) ccw projected
  line L85 (231.8, -18) -> (231.8, -22) projected
  arc A57 (333.1, -102) -> (337.5, -102) centre (335.3, -102) ccw projected
  line L86 (333.1, -102) -> (333.1, -98) projected
  arc A58 (337.5, -98) -> (333.1, -98) centre (335.3, -98) ccw projected
  line L87 (337.5, -98) -> (337.5, -102) projected
  arc A59 (347.5, -102) -> (351.9, -102) centre (349.7, -102) ccw projected
  line L88 (347.5, -102) -> (347.5, -98) projected
  arc A60 (351.9, -98) -> (347.5, -98) centre (349.7, -98) ccw projected
  line L89 (351.9, -98) -> (351.9, -102) projected
  arc A61 (337.5, -18) -> (333.1, -18) centre (335.3, -18) ccw projected
  line L90 (337.5, -18) -> (337.5, -22) projected
  arc A62 (333.1, -22) -> (337.5, -22) centre (335.3, -22) ccw projected
  line L91 (333.1, -22) -> (333.1, -18) projected
  arc A63 (351.9, -18) -> (347.5, -18) centre (349.7, -18) ccw projected
  line L92 (351.9, -18) -> (351.9, -22) projected
  arc A64 (347.5, -22) -> (351.9, -22) centre (349.7, -22) ccw projected
  line L93 (347.5, -22) -> (347.5, -18) projected
  circle A65 centre (253.534, -95) radius 2 projected
  circle A66 centre (156.066, -95) radius 2 projected
  circle A67 centre (156.066, -25) radius 2 projected
  line L94 (0, -90.2572) -> (13.6, -82.4053) projected
  line L95 (355, -4.1) -> (0, -4.1) projected
  point P0 (276.8, -60)
  point P1 (249.3, -60)
  point P2 (276.8, -15)
  point P3 (14.7, -40)
  dimension "d140" = 5
  dimension "d141" = 90
  dimension "d147" = 55
  constraints: 14 end point, 8 point on circle, 8 tangent, 4 centre point, 3 equal radius, 3 horizontal alignment, 3 midpoint, 2 horizontal, 2 parallel, 2 perpendicular, 1 vertical, 1 vertical alignment, 1 other
  measures "d140" radius of A14
  measures "d141" distance between parallel lines of L30 L28
  measures "d147" distance between parallel lines of L31 L29
sheet face with bend "Cara3" sketch "Boceto5" thickness 4 toward (0, 0, 1) bend radius 0.1 relief tear relief width 4 relief depth 2 contours L95 L3 L38 L4 L36 A5 L11 A4 L32 | L18 A8 L16 A7 L15 L40 | L22 A10 L24 A12 L27 L50 | L31 A35 | A39 L29 | L31 A37 | A34 L29
bend "Doblez4"
ref_plane "Plano de trabajo1" through (276.8, 60, -56) normal (0, 0, 1) x (1, 0, 0)
mirror "Simetría1" about plane through (276.8, 60, -56) normal (0, 0, 1) of "Pliegue1", "Pliegue2"
sketch "Boceto6" plane through (-78.2, -56, -0.1) normal (0, 1, 0) x (1, 0, 0)
  arc A0 (14.6, 76.4) -> (10.4, 76.4) centre (12.5, 76.4) ccw projected
  arc A1 (10.4, 35.4) -> (14.6, 35.4) centre (12.5, 35.4) ccw projected
  line L0 (14.6, 35.4) -> (14.6, 76.4)
  line L1 (10.4, 76.4) -> (10.4, 35.4)
  arc A2 (17.5, 93.9) -> (21.7, 93.9) centre (19.6, 93.9) ccw projected
  line L2 (17.5, 93.9) -> (17.5, 97.9) projected
  arc A3 (21.7, 97.9) -> (17.5, 97.9) centre (19.6, 97.9) ccw projected
  line L3 (21.7, 97.9) -> (21.7, 93.9) projected
  arc A4 (7.5, 97.9) -> (3.3, 97.9) centre (5.4, 97.9) ccw projected
  line L4 (7.5, 97.9) -> (7.5, 93.9) projected
  arc A5 (3.3, 93.9) -> (7.5, 93.9) centre (5.4, 93.9) ccw projected
  line L5 (3.3, 93.9) -> (3.3, 97.9) projected
  arc A6 (127.2, 97.9) -> (123, 97.9) centre (125.1, 97.9) ccw projected
  line L6 (127.2, 97.9) -> (127.2, 93.9) projected
  arc A7 (123, 93.9) -> (127.2, 93.9) centre (125.1, 93.9) ccw projected
  line L7 (123, 93.9) -> (123, 97.9) projected
  arc A8 (113, 97.9) -> (108.8, 97.9) centre (110.9, 97.9) ccw projected
  line L8 (113, 97.9) -> (113, 93.9) projected
  arc A9 (108.8, 93.9) -> (113, 93.9) centre (110.9, 93.9) ccw projected
  line L9 (108.8, 93.9) -> (108.8, 97.9) projected
  arc A10 (333.3, 93.9) -> (337.5, 93.9) centre (335.4, 93.9) ccw projected
  line L10 (333.3, 93.9) -> (333.3, 97.9) projected
  arc A11 (337.5, 97.9) -> (333.3, 97.9) centre (335.4, 97.9) ccw projected
  line L11 (337.5, 97.9) -> (337.5, 93.9) projected
  arc A12 (347.5, 93.9) -> (351.7, 93.9) centre (349.6, 93.9) ccw projected
  line L12 (347.5, 93.9) -> (347.5, 97.9) projected
  arc A13 (351.7, 97.9) -> (347.5, 97.9) centre (349.6, 97.9) ccw projected
  line L13 (351.7, 97.9) -> (351.7, 93.9) projected
  line L14 (355, 111.8) -> (0, 111.8) construction
  line L15 (0, 111.8) -> (0, 56.15) projected
  line L16 (0, 56.15) -> (10.4, 56.15) projected
  line L17 (10.4, 56.15) -> (10.4, 76.4) projected
  arc A14 (14.6, 76.4) -> (10.4, 76.4) centre (12.5, 76.4) ccw projected
  line L18 (14.6, 76.4) -> (14.6, 56.15) projected
  line L19 (14.6, 56.15) -> (115.9, 56.15) construction
  line L20 (115.9, 56.15) -> (115.9, 76.4) construction
  arc A15 (120.1, 76.4) -> (115.9, 76.4) centre (118, 76.4) ccw projected
  line L21 (120.1, 76.4) -> (120.1, 56.15) construction
  line L22 (120.1, 56.15) -> (130.8, 56.15) construction
  line L23 (130.8, 56.15) -> (130.8, 79.9) construction
  arc A16 (142.8, 91.9) -> (130.8, 79.9) centre (142.8, 79.9) ccw projected
  line L24 (142.8, 91.9) -> (318, 91.9) construction
  arc A17 (330, 79.9) -> (318, 91.9) centre (318, 79.9) ccw projected
  line L25 (330, 79.9) -> (330, 56.15) projected
  line L26 (330, 56.15) -> (340.4, 56.15) projected
  line L27 (340.4, 56.15) -> (340.4, 76.4) construction
  arc A18 (341.45, 78.2187) -> (340.4, 76.4) centre (342.5, 76.4) ccw projected
  line L28 (341.45, 78.2187) -> (355, 86.0417) construction
  line L29 (355, 86.0417) -> (355, 111.8) construction
  arc A19 (347.5, 13.9) -> (351.7, 13.9) centre (349.6, 13.9) ccw projected
  line L30 (347.5, 13.9) -> (347.5, 17.9) projected
  arc A20 (351.7, 17.9) -> (347.5, 17.9) centre (349.6, 17.9) ccw projected
  line L31 (351.7, 17.9) -> (351.7, 13.9) projected
  arc A21 (333.3, 13.9) -> (337.5, 13.9) centre (335.4, 13.9) ccw projected
  line L32 (333.3, 13.9) -> (333.3, 17.9) projected
  arc A22 (337.5, 17.9) -> (333.3, 17.9) centre (335.4, 17.9) ccw projected
  line L33 (337.5, 17.9) -> (337.5, 13.9) projected
  arc A23 (113, 17.9) -> (108.8, 17.9) centre (110.9, 17.9) ccw projected
  line L34 (113, 17.9) -> (113, 13.9) projected
  arc A24 (108.8, 13.9) -> (113, 13.9) centre (110.9, 13.9) ccw projected
  line L35 (108.8, 13.9) -> (108.8, 17.9) projected
  arc A25 (127.2, 17.9) -> (123, 17.9) centre (125.1, 17.9) ccw projected
  line L36 (127.2, 17.9) -> (127.2, 13.9) projected
  arc A26 (123, 13.9) -> (127.2, 13.9) centre (125.1, 13.9) ccw projected
  line L37 (123, 13.9) -> (123, 17.9) projected
  arc A27 (21.7, 17.9) -> (17.5, 17.9) centre (19.6, 17.9) ccw projected
  line L38 (21.7, 17.9) -> (21.7, 13.9) projected
  arc A28 (17.5, 13.9) -> (21.7, 13.9) centre (19.6, 13.9) ccw projected
  line L39 (17.5, 13.9) -> (17.5, 17.9) projected
  arc A29 (7.5, 17.9) -> (3.3, 17.9) centre (5.4, 17.9) ccw projected
  line L40 (7.5, 17.9) -> (7.5, 13.9) projected
  arc A30 (3.3, 13.9) -> (7.5, 13.9) centre (5.4, 13.9) ccw projected
  line L41 (3.3, 13.9) -> (3.3, 17.9) projected
  line L42 (120.1, 55.65) -> (120.1, 35.4) construction
  arc A31 (115.9, 35.4) -> (120.1, 35.4) centre (118, 35.4) ccw projected
  line L43 (115.9, 35.4) -> (115.9, 55.65) construction
  line L44 (115.9, 55.65) -> (14.6, 55.65) construction
  line L45 (14.6, 55.65) -> (14.6, 35.4) projected
  arc A32 (10.4, 35.4) -> (14.6, 35.4) centre (12.5, 35.4) ccw projected
  line L46 (10.4, 35.4) -> (10.4, 55.65) projected
  line L47 (10.4, 55.65) -> (0, 55.65) projected
  line L48 (0, 55.65) -> (0, 0) projected
  line L49 (355, 0) -> (0, 0) construction
  line L50 (355, 0) -> (355, 25.7583) construction
  line L51 (355, 25.7583) -> (341.45, 33.5813) construction
  arc A33 (340.4, 35.4) -> (341.45, 33.5813) centre (342.5, 35.4) ccw projected
  line L52 (340.4, 35.4) -> (340.4, 55.65) construction
  line L53 (340.4, 55.65) -> (330, 55.65) projected
  line L54 (330, 55.65) -> (330, 31.9) projected
  arc A34 (318, 19.9) -> (330, 31.9) centre (318, 31.9) ccw projected
  line L55 (318, 19.9) -> (142.8, 19.9) construction
  arc A35 (130.8, 31.9) -> (142.8, 19.9) centre (142.8, 31.9) ccw projected
  line L56 (130.8, 31.9) -> (130.8, 55.65) construction
  line L57 (130.8, 55.65) -> (120.1, 55.65) construction
  arc A36 (344.6, 76.4) -> (341.45, 78.2187) centre (342.5, 76.4) ccw
  line L58 (344.6, 76.4) -> (344.6, 35.4)
  arc A37 (341.45, 33.5813) -> (344.6, 35.4) centre (342.5, 35.4) ccw
  arc A38 (115.9, 35.4) -> (120.1, 35.4) centre (118, 35.4) ccw projected
  line L59 (115.9, 35.4) -> (115.9, 76.4)
  line L60 (120.1, 35.4) -> (120.1, 76.4)
  line L61 (340.4, 76.4) -> (340.4, 35.4)
  point P0 (78.2, -0.1)
  constraints: 12 end point, 8 tangent, 5 vertical, 4 point on circle, 2 centre point, 1 concentric, 1 parallel
extrude "Extrusión5" cut sketch "Boceto6" against normal blind 10
